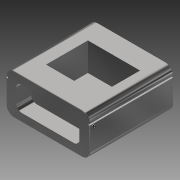
# Autodesk Inventor part: Body Part
Saved by Autodesk Inventor 2015 (Build 190159000, 159)
## iProperties
Created: 2015-01-12
Part Number: Body Part
Material: Generic
Document SubType Name: Modeling
Designer: PLTW-Stu-02
Density: 1 g/cm^3
Appearance: Steel - Polished
Author: PLTW-Stu-02
Autodesk Inventor part; units mm, degrees
ref_plane "YZ Plane" through (0, 0, 0) normal (1, 0, 0) x (0, 1, 0)
ref_plane "XZ Plane" through (0, 0, 0) normal (0, 1, 0) x (-1, 0, 0)
ref_plane "XY Plane" through (0, 0, 0) normal (0, 0, 1) x (1, 0, 0)
sketch "Sketch1" plane through (0, 0, 0) normal (0, 0, 1) x (1, 0, 0)
  line L0 (-16.6217, 13.0116) -> (48.6563, 13.0116)
  line L1 (56.2763, 5.3916) -> (56.2763, -18.2304)
  line L2 (48.6563, -25.8504) -> (-16.6217, -25.8504)
  line L3 (-24.2417, -18.2304) -> (-24.2417, 5.3916)
  arc A0 (-21.0667, 13.0116) -> (-24.2417, 9.8366) centre (-21.0667, 9.8366) ccw
  arc A1 (-16.6217, 13.0116) -> (-24.2417, 5.3916) centre (-16.6217, 5.3916) ccw
  arc A2 (56.2763, 5.3916) -> (48.6563, 13.0116) centre (48.6563, 5.3916) ccw
  arc A3 (48.6563, -25.8504) -> (56.2763, -18.2304) centre (48.6563, -18.2304) ccw
  arc A4 (-24.2417, -18.2304) -> (-16.6217, -25.8504) centre (-16.6217, -18.2304) ccw
  point P0 (0, 0)
  point P1 (56.2763, -25.8504)
  point P2 (56.2763, 13.0116)
  point P3 (-24.2417, -25.8504)
  dimension "d0" = 80.518
  dimension "d1" = 38.862
  dimension "d2" = 3.175
  dimension "d3" = 7.62
  constraints: 10 point on circle, 10 tangent, 8 end point, 8 point on line, 5 centre point, 3 equal radius, 2 parallel, 1 horizontal, 1 perpendicular
  measures "d0" distance of point (56.276, -25.85) point (-24.242, -25.85)
  measures "d1" distance of point (56.276, 13.012) point (56.276, -25.85)
  measures "d2" radius of A0
  measures "d3" radius of A1
extrude "Extrusion1" add sketch "Sketch1" along normal blind 80.518
sketch "Sketch2" plane through (-16.6217, 13.0116, 0) normal (0, 1, 0) x (1, 0, 0)
  line L0 (72.898, 0) -> (72.898, -80.518) projected
  line L1 (60.198, -59.69) -> (9.906, -59.69)
  line L2 (9.906, -59.69) -> (9.906, -19.304)
  line L3 (9.906, -19.304) -> (60.198, -19.304)
  line L4 (60.198, -19.304) -> (60.198, -59.69)
  point P0 (16.6217, 0)
  dimension "d27" = 50.292
  constraints: 8 end point, 2 parallel, 1 horizontal, 1 perpendicular
  measures "d27" distance of L2.end L3.end
extrude "Extrusion2" cut sketch "Sketch2" against normal blind 27.178
sketch "Sketch4" plane through (0, 0, 80.518) normal (0, 0, 1) x (1, 0, 0)
  arc A0 (56.2763, 5.3916) -> (48.6563, 13.0116) centre (48.6563, 5.3916) ccw projected
  arc A1 (-16.6217, 13.0116) -> (-24.2417, 5.3916) centre (-16.6217, 5.3916) ccw projected
  line L0 (41.2903, 5.3916) -> (-9.5097, 5.3916)
  line L1 (-14.5897, 0.3116) -> (-14.5897, -13.1504)
  line L2 (-9.5097, -18.2304) -> (41.2903, -18.2304)
  line L3 (46.3703, -13.1504) -> (46.3703, 0.3116)
  arc A2 (-9.5097, 5.3916) -> (-14.5897, 0.3116) centre (-9.5097, 0.3116) ccw
  arc A3 (-14.5897, -13.1504) -> (-9.5097, -18.2304) centre (-9.5097, -13.1504) ccw
  arc A4 (41.2903, -18.2304) -> (46.3703, -13.1504) centre (41.2903, -13.1504) ccw
  arc A5 (46.3703, 0.3116) -> (41.2903, 5.3916) centre (41.2903, 0.3116) ccw
  point P0 (0, 0)
  point P1 (43.0449, 12.5609)
  point P2 (-14.5897, -18.2304)
  point P3 (-14.5897, 5.3916)
  point P4 (46.3703, -18.2304)
  dimension "d39" = 60.96
  dimension "d40" = 23.622
  dimension "d41" = 5.08
  constraints: 8 end point, 8 point on circle, 8 tangent, 6 point on line, 4 centre point, 3 equal radius, 2 parallel, 1 horizontal, 1 perpendicular
  measures "d39" distance of point (46.37, -18.23) point (-14.59, -18.23)
  measures "d40" distance of point (-14.59, -18.23) point (-14.59, 5.392)
  measures "d41" radius of A2
extrude "Extrusion3" cut sketch "Sketch4" against normal blind 14.478
sketch "Sketch5" plane through (0, 0, 80.518) normal (0, 0, 1) x (1, 0, 0)
  line L0 (56.2763, 5.3916) -> (54.7523, 5.3916)
  line L1 (54.7523, 5.3916) -> (54.7523, 3.8676)
  line L2 (54.7523, 3.8676) -> (56.2763, 3.8676)
  line L3 (56.2763, 3.8676) -> (56.2763, 5.3916)
  point P0 (0, 0)
  constraints: 8 end point, 2 parallel, 1 horizontal, 1 perpendicular
extrude "Extrusion4" cut sketch "Sketch5" against normal through all
sketch "Sketch7" plane through (0, 0, 0) normal (0, 0, -1) x (-1, 0, 0)
  line L0 (15.6057, 6.1536) -> (-47.8943, 6.1536)
  line L1 (-47.8943, 6.1536) -> (-47.8943, -19.2464)
  line L2 (-47.8943, -19.2464) -> (15.6057, -19.2464)
  line L3 (15.6057, -19.2464) -> (15.6057, 6.1536)
  point P0 (0, 0)
  dimension "d59" = 25.4
  dimension "d60" = 63.5
  constraints: 8 end point, 2 parallel, 1 horizontal, 1 perpendicular
  measures "d59" distance of L1.end L0.end
  measures "d60" distance of L1.end L2.end
extrude "Extrusion5" cut sketch "Sketch7" against normal blind 14.478
sketch "Sketch8" plane through (56.2763, -18.2304, 80.518) normal (1, 0, 0) x (0, 0, -1)
  line L0 (1.7031, 21.4246) -> (7.948, 21.4246) construction
  line L1 (7.948, 21.4246) -> (7.948, 17.7638) construction
  line L2 (7.948, 17.7638) -> (1.7031, 17.7638) construction
  line L3 (1.7031, 17.7638) -> (1.7031, 21.4246) construction
  spline S0 degree 2 poles (4.0499, 21.1728) (4.0499, 21.1041) (4.0384, 21.0068) (4.0155, 20.9495) (3.9783, 20.9209) (3.9583, 20.9209) knots 0 0 0 1 2 3 4 4 4
  line L4 (3.9583, 20.9209) -> (3.1999, 20.9209)
  line L5 (3.1999, 20.9209) -> (3.1999, 18.4739)
  spline S1 degree 2 poles (3.1999, 18.4739) (3.1999, 18.451) (3.1684, 18.4138) (3.0997, 18.3909) (2.9795, 18.3766) (2.8908, 18.3766) knots 0 0 0 1 2 3 4 4 4
  spline S2 degree 2 poles (2.8908, 18.3766) (2.8021, 18.3766) (2.6819, 18.3909) (2.6132, 18.4138) (2.5817, 18.451) (2.5817, 18.4739) knots 0 0 0 1 2 3 4 4 4
  line L6 (2.5817, 18.4739) -> (2.5817, 20.9209)
  line L7 (2.5817, 20.9209) -> (1.8233, 20.9209)
  spline S3 degree 2 poles (1.8233, 20.9209) (1.8004, 20.9209) (1.766, 20.9495) (1.7431, 21.0068) (1.7317, 21.1041) (1.7317, 21.1728) knots 0 0 0 1 2 3 4 4 4
  spline S4 degree 2 poles (1.7317, 21.1728) (1.7317, 21.2415) (1.7431, 21.3416) (1.766, 21.3989) (1.8004, 21.4246) (1.8233, 21.4246) knots 0 0 0 1 2 3 4 4 4
  line L8 (1.8233, 21.4246) -> (3.9583, 21.4246)
  spline S5 degree 2 poles (3.9583, 21.4246) (3.9783, 21.4246) (4.0155, 21.3989) (4.0384, 21.3416) (4.0499, 21.2415) (4.0499, 21.1728) knots 0 0 0 1 2 3 4 4 4
  spline S6 degree 2 poles (5.3089, 19.287) (5.3089, 19.1877) (5.2887, 18.9723) (5.2314, 18.7661) (5.1306, 18.5816) (4.9725, 18.4421) (4.7446, 18.3615) (4.5896, 18.3615) knots 0 0 0 1 2 3 4 5 6 6 6
  spline S7 degree 2 poles (4.5896, 18.3615) (4.5353, 18.3615) (4.4268, 18.377) (4.3369, 18.4002) (4.2749, 18.425) (4.247, 18.4514) (4.2346, 18.5025) (4.2346, 18.5475) knots 0 0 0 1 2 3 4 5 6 6 6
  spline S8 degree 2 poles (4.2346, 18.5475) (4.2346, 18.5894) (4.2377, 18.6405) (4.2501, 18.6684) (4.2671, 18.6777) (4.278, 18.6777) knots 0 0 0 1 2 3 4 4 4
  spline S9 degree 2 poles (4.278, 18.6777) (4.2935, 18.6777) (4.3493, 18.6591) (4.4284, 18.6359) (4.5307, 18.6188) (4.5927, 18.6188) knots 0 0 0 1 2 3 4 4 4
  spline S10 degree 2 poles (4.5927, 18.6188) (4.6996, 18.6188) (4.8469, 18.6948) (4.9384, 18.825) (4.9818, 18.9955) (4.9849, 19.0901) knots 0 0 0 1 2 3 4 4 4
  spline S11 degree 2 poles (4.9849, 19.0901) (4.926, 19.0529) (4.7617, 18.9986) (4.6547, 18.9986) knots 0 0 0 1 2 2 2
  spline S12 degree 2 poles (4.6547, 18.9986) (4.5229, 18.9986) (4.34, 19.0668) (4.2268, 19.197) (4.1741, 19.3815) (4.1741, 19.4993) knots 0 0 0 1 2 3 4 4 4
  spline S13 degree 2 poles (4.1741, 19.4993) (4.1741, 19.6218) (4.2485, 19.8295) (4.3927, 19.9799) (4.6082, 20.0636) (4.7508, 20.0636) knots 0 0 0 1 2 3 4 4 4
  spline S14 degree 2 poles (4.7508, 20.0636) (4.8655, 20.0636) (5.0376, 20.0109) (5.1601, 19.9117) (5.2422, 19.7706) (5.2903, 19.597) (5.3089, 19.397) (5.3089, 19.287) knots 0 0 0 1 2 3 4 5 6 6 6
  spline S15 degree 2 poles (4.9771, 19.3335) (4.9771, 19.4699) (4.9461, 19.6513) (4.8857, 19.7613) (4.7942, 19.8063) (4.7322, 19.8063) knots 0 0 0 1 2 3 4 4 4
  spline S16 degree 2 poles (4.7322, 19.8063) (4.6733, 19.8063) (4.5865, 19.7644) (4.5291, 19.6885) (4.5012, 19.5846) (4.5012, 19.5226) knots 0 0 0 1 2 3 4 4 4
  spline S17 degree 2 poles (4.5012, 19.5226) (4.5012, 19.4559) (4.526, 19.3536) (4.5772, 19.2854) (4.6609, 19.2529) (4.7213, 19.2529) knots 0 0 0 1 2 3 4 4 4
  spline S18 degree 2 poles (4.7213, 19.2529) (4.7958, 19.2529) (4.926, 19.2978) (4.9771, 19.3335) knots 0 0 0 1 2 2 2
  point P0 (80.518, 18.2304)
  constraints: 2 other
emboss "Emboss2" sketch "Sketch8" operation add depth 0.508 direction (-1, 0, 0)
sketch "Sketch9" plane through (-24.2417, -18.2304, 0) normal (-1, 0, 0) x (0, 0, 1)
  line L0 (80.518, 23.622) -> (0, 23.622)
  line L1 (0, 23.622) -> (0, 22.098)
  line L2 (0, 22.098) -> (80.518, 22.098)
  line L3 (80.518, 22.098) -> (80.518, 23.622)
  point P0 (0, 18.2304)
  constraints: 8 end point, 2 parallel, 1 horizontal, 1 perpendicular
extrude "Extrusion6" cut sketch "Sketch9" against normal blind 1.524
chamfer "Chamfer1" distance 0.254 angle 45 3 edges at (16.0173, 13.0116, 80.518) (-22.0098, 10.7798, 80.518) (54.0445, 10.7798, 80.518)
chamfer "Chamfer2" distance 0.254 angle 45 8 edges at (16.0173, 12.7576, 80.518) (53.8649, 10.6002, 80.518) (-21.8302, 10.6002, 80.518) (56.2763, -7.1814, 80.518) (54.0445, -23.6185, 80.518) (16.0173, -25.8504, 80.518) (-22.0098, -23.6185, 80.518) (-24.2417, -7.1814, 80.518)
chamfer "Chamfer3" distance 0.254 angle 45 3 edges at (54.0445, 10.7798, 0) (16.0173, 13.0116, 0) (-22.0098, 10.7798, 0)
chamfer "Chamfer4" distance 0.254 angle 45 5 edges at (56.2763, -7.1814, 0) (54.0445, -23.6185, 0) (16.0173, -25.8504, 0) (-22.0098, -23.6185, 0) (-24.2417, -7.1814, 0)
body "Solid1"
